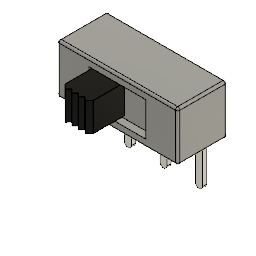
SPDT MSHS1105 APEM v1 (Autodesk Fusion 360 design; units mm, degrees)
Autodesk Fusion 360 part; units mm, degrees
note: some values were not read from the file. Chosen so that the rebuilt part matches the saved one: which face or edge a step refers to.
sketch "Sketch1" plane through (0, 0, 0) normal (0, 1, 0) x (1, 0, 0)
  line L0 (4.25, 1.75) -> (-4.25, 1.75)
  line L1 (-4.25, 1.75) -> (-4.25, -1.75)
  line L2 (-4.25, -1.75) -> (4.25, -1.75)
  line L3 (4.25, -1.75) -> (4.25, 1.75)
  line L4 (4.25, 1.75) -> (-4.25, -1.75) construction
  line L5 (-4.25, 1.75) -> (4.25, -1.75) construction
  dimension "d1" = 8.5
  dimension "d2" = 3.5
extrude "Extrude1" add sketch "Sketch1" along normal blind 3.5 makes body 1
sketch "Sketch3" plane through (0, 0, 0) normal (0, -1, 0) x (1, 0, 0)
  line L0 (4.25, -1.75) -> (4.25, 1.75)
  line L1 (4.25, 1.75) -> (-4.25, 1.75)
  line L2 (-4.25, 1.75) -> (-4.25, -1.75)
  line L3 (-4.25, -1.75) -> (4.25, -1.75)
  line L4 (2.0048, -1.2033) -> (-2.0048, -1.2033)
  line L5 (-2.0048, -1.2033) -> (-2.0048, 1.2033)
  line L6 (-2.0048, 1.2033) -> (2.0048, 1.2033)
  line L7 (2.0048, 1.2033) -> (2.0048, -1.2033)
  line L8 (2.0048, -1.2033) -> (-2.0048, 1.2033) construction
  line L9 (-2.0048, -1.2033) -> (2.0048, 1.2033) construction
  line L10 (0.0073, -1.0293) -> (-1.9927, -1.0293)
  line L11 (-1.9927, -1.0293) -> (-1.9927, 1)
  line L12 (-1.9927, 1) -> (0.0073, 1)
  line L13 (0.0073, 1) -> (0.0073, -1.0293)
  dimension "d7" = 2
extrude "Extrude2" cut sketch "Sketch3" against normal blind 0.5 contours L4 L5 L6 L7 bodies 1
extrude "Extrude3" add 1 faces at (-0.6593, 0, 0.3236) along direction (0, -1, 0) blind 2 and the other way blind 0.5 separate body on bodies 1 makes body 2
sketch "Sketch4" plane through (0, 3.5, 0) normal (0, 1, 0) x (-1, 0, 0)
  line L0 (-4.25, 1.75) -> (-4.25, -1.75)
  line L1 (-4.25, -1.75) -> (4.25, -1.75)
  line L2 (4.25, -1.75) -> (4.25, 1.75)
  line L3 (4.25, 1.75) -> (-4.25, 1.75)
  line L4 (-2.8873, -1.75) -> (-2.8873, -2.8)
  line L5 (-2.8873, -2.8) -> (-2.8, -2.9)
  line L6 (-2.8, -2.9) -> (-2.8, -5.3)
  arc A0 (-2.8, -5.3) -> (-2.3, -5.3) centre (-2.55, -5.3) ccw
  line L7 (-2.3, -5.3) -> (-2.3, -2.9)
  line L8 (-2.3, -2.9) -> (-2.2, -2.8)
  line L9 (-2.2, -2.8) -> (-2.2, -1.75)
  line L10 (-2.8873, -1.75) -> (-2.2, -1.75)
  line L11 (-0.3873, -1.75) -> (0.3, -1.75)
  line L12 (-0.3873, -1.75) -> (-0.3873, -2.8)
  line L13 (-0.3873, -2.8) -> (-0.3, -2.9)
  line L14 (-0.3, -2.9) -> (-0.3, -5.3)
  arc A1 (-0.3, -5.3) -> (0.2, -5.3) centre (-0.05, -5.3) ccw
  line L15 (0.2, -5.3) -> (0.2, -2.9)
  line L16 (0.2, -2.9) -> (0.3, -2.8)
  line L17 (0.3, -2.8) -> (0.3, -1.75)
  line L18 (2.1127, -1.75) -> (2.8, -1.75)
  line L19 (2.1127, -1.75) -> (2.1127, -2.8)
  line L20 (2.1127, -2.8) -> (2.2, -2.9)
  line L21 (2.2, -2.9) -> (2.2, -5.3)
  arc A2 (2.2, -5.3) -> (2.7, -5.3) centre (2.45, -5.3) ccw
  line L22 (2.7, -5.3) -> (2.7, -2.9)
  line L23 (2.7, -2.9) -> (2.8, -2.8)
  line L24 (2.8, -2.8) -> (2.8, -1.75)
  dimension "d14" = 0.5
  dimension "d17" = 5
  dimension "d18" = 0
  measures "d14" distance of L6 L7
extrude "Extrude4" add sketch "Sketch4" against normal blind 0.3 separate body contours L1 L4 L5 L6 A0 L7 L8 L9 L10 | L1 L18 L19 L20 L21 A2 L22 L23 L24 | L1 L11 L12 L13 L14 A1 L15 L16 L17 makes body 3 at (2.6582, 3.5, -2.1) makes body 4 at (0.1582, 3.5, -2.1) makes body 5 at (-2.3418, 3.5, -2.1)
sketch "Sketch5" plane through (0, 0, 1) normal (0, 0, 1) x (-1, 0, 0)
  line L0 (1.9927, -0.5) -> (1.9927, 2)
  line L1 (1.9927, 2) -> (-0.0073, 2)
  line L2 (-0.0073, 2) -> (-0.0073, -0.5)
  line L3 (-0.0073, -0.5) -> (1.9927, -0.5)
  line L4 (1.9927, 2) -> (-0.0073, 2)
  line L5 (-0.0073, 2) -> (-0.0073, 1.6948)
  line L6 (-0.0073, 1.6948) -> (1.9927, 1.6948)
  line L7 (1.9927, 1.6948) -> (1.9927, 2)
  line L8 (1.9927, 1.6948) -> (1.6839, 2)
  line L9 (1.6839, 2) -> (1.3822, 1.6948)
  line L10 (1.526, 1.6948) -> (1.2173, 2)
  line L11 (1.2173, 2) -> (0.9155, 1.6948)
  line L12 (1.0593, 1.6948) -> (0.7506, 2)
  line L13 (0.7506, 2) -> (0.4488, 1.6948)
  line L14 (0.5927, 1.6948) -> (0.2839, 2)
  line L15 (0.2839, 2) -> (-0.0178, 1.6948)
  dimension "d23" = -1.4
  dimension "d24" = 0
extrude "Extrude5" cut sketch "Sketch5" against normal blind 2.5 contours L0 L1 L4 L7 L8 | L1 L4 L9 L10 | L1 L4 L11 L12 | L1 L2 L4 L5 L15 | L1 L4 L13 L14 bodies 2
delete_face "DeleteFace1" 5 faces at (0.0073, 0.1667, 0.3236) (-1.326, 0.1667, 1) (-1.9927, 0.1667, -0.3529) (-0.6593, 0.1667, -1.0293) (-0.6593, 0, 0.3236) on bodies 1
fillet "Fillet1" radius 0.15 12 edges at (0, 0, 1.75) (4.25, 1.75, 1.75) (0, 3.5, 1.75) (-4.25, 1.75, 1.75) (4.25, 0, 0) (4.25, 3.5, 0) (4.25, 1.75, -1.75) (0, 0, -1.75) (-4.25, 0, 0) (-4.25, 3.5, 0) (-4.25, 1.75, -1.75) (0, 3.5, -1.75) on bodies 1
